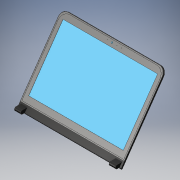
# Autodesk Inventor part: MONITOR
Saved by Autodesk Inventor 2025 (Build 290162000, 162)
## iProperties
Created: 2017-02-17
Part Number: MONITOR
Material: Generic
Document SubType Name: Modeling
Designer: Ali
Density: 1 g/cm^3
Appearance: Default
Author: Ali
Autodesk Inventor part; units mm, degrees
ref_plane "XZ Plane" through (0, 0, 0) normal (0, 1, 0) x (-1, 0, 0)
ref_plane "XY Plane" through (0, 0, 0) normal (0, 0, 1) x (1, 0, 0)
sketch "Sketch1" plane through (0, 0, 0) normal (0, 0, 1) x (1, 0, 0)
  line L0 (-145, 250) -> (145, 250)
  line L1 (165, 230) -> (165, 0)
  line L2 (165, 0) -> (-165, 0)
  line L3 (-165, 0) -> (-165, 230)
  arc A0 (-145, 250) -> (-165, 230) centre (-145, 230) ccw
  arc A1 (165, 230) -> (145, 250) centre (145, 230) ccw
  point P0 (0, 0)
  point P1 (165, 250)
  dimension "d2" = 330
  dimension "d3" = 250
  dimension "d4" = 20
  constraints: 8 end point, 4 point on circle, 4 tangent, 2 centre point, 2 parallel, 2 point on line, 1 equal radius, 1 horizontal, 1 perpendicular
  measures "d2" distance of L1.end L2.end
  measures "d3" distance of point (165, 250) L1.end
  measures "d4" radius of A0
extrude "MONITOR" add sketch "Sketch1" along normal blind 5
sketch "Sketch2" plane through (0, 0, 5) normal (0, 0, 1) x (1, 0, 0)
  line L0 (150, 40) -> (-150, 40)
  line L1 (-150, 40) -> (-150, 230)
  line L2 (-150, 230) -> (150, 230)
  line L3 (150, 230) -> (150, 40)
  dimension "d9" = 300
  dimension "d10" = 190
  constraints: 8 end point, 2 parallel, 1 horizontal, 1 perpendicular
  measures "d9" distance of L1.end L2.end
  measures "d10" distance of L0.end L1.end
extrude "SCREEN" cut sketch "Sketch2" against normal blind 0.5
sketch "Sketch3" plane through (0, 0, 5) normal (0, 0, 1) x (1, 0, 0)
  circle A0 centre (0, 240) radius 2.5
  point P0 (0, 0)
  constraints: 1 centre point
sketch "Sketch4" plane through (0, 240, 5.25) normal (0, 0, 1) x (1, 0, 0)
  point P0 (0, -240)
  point P1 (0, 0)
extrude "CAMERA" add sketch "Sketch3" along normal blind 0.25
extrude "CAMERA" add sketch "Sketch3" along normal blind 0.25
hole "CAMERA " at (0, 240, 5.25) direction (0, 0, -1) diameter 1 depth 0.1 tip angle 118
sketch "Sketch5" plane through (0, 0, 5) normal (0, 0, 1) x (1, 0, 0)
  point P0 (0, 0)
  point P1 (15, 240)
  point P2 (30, 240)
  point P3 (-15, 240)
hole "AESTHETICS" at (15, 240, 5) at (30, 240, 5) at (-15, 240, 5) direction (0, 0, -1) diameter 1 depth 0.1 tip angle 118
sketch "Sketch6" plane through (0, 0, 5) normal (0, 0, 1) x (1, 0, 0)
  line L0 (164.5, 20) -> (-164.5, 20)
  line L1 (-164.5, 20) -> (-164.5, 229)
  line L2 (-144, 249.5) -> (144, 249.5)
  line L3 (164.5, 229) -> (164.5, 20)
  arc A0 (-144, 249.5) -> (-164.5, 229) centre (-144, 229) ccw
  arc A1 (164.5, 229) -> (144, 249.5) centre (144, 229) ccw
  point P0 (-164.5, 249.5)
  point P1 (164.5, 249.5)
  dimension "d36" = 229.5
  dimension "d37" = 20.5
  dimension "d38" = 329
  constraints: 8 end point, 4 point on circle, 4 point on line, 4 tangent, 2 centre point, 2 parallel, 1 equal radius, 1 horizontal, 1 perpendicular
  measures "d36" distance of L0.end point (-164.5, 249.5)
  measures "d37" radius of A0
  measures "d38" distance of L0.start L0.end
extrude "SIDE BAND" add sketch "Sketch6" along normal blind 0.15
sketch "Sketch7" plane through (0, 0, 5) normal (0, 0, 1) x (1, 0, 0)
  line L0 (161.5, 23) -> (-161.5, 23)
  line L1 (-161.5, 23) -> (-161.5, 223)
  line L2 (-138, 246.5) -> (138, 246.5)
  line L3 (161.5, 223) -> (161.5, 23)
  arc A0 (-138, 246.5) -> (-161.5, 223) centre (-138, 223) ccw
  arc A1 (161.5, 223) -> (138, 246.5) centre (138, 223) ccw
  point P0 (-161.5, 246.5)
  point P1 (161.5, 246.5)
  dimension "d47" = 323
  dimension "d48" = 223.5
  dimension "d49" = 23.5
  constraints: 8 end point, 4 point on circle, 4 point on line, 4 tangent, 2 centre point, 2 parallel, 1 equal radius, 1 horizontal, 1 perpendicular
  measures "d47" distance of point (-161.5, 246.5) point (161.5, 246.5)
  measures "d48" distance of L0.end point (-161.5, 246.5)
  measures "d49" radius of A0
extrude "SIDE BAND 1" cut sketch "Sketch7" along normal blind 0.15
sketch "Sketch8" plane through (165, 0, 0) normal (1, 0, 0) x (0, 0, -1)
  line L0 (0, 0) -> (-5, 0)
  line L1 (-5, 0) -> (-5, 2.251)
  line L2 (-5, 2.251) -> (0, 2.251)
  line L3 (0, 2.251) -> (0, 0)
  constraints: 8 end point, 2 parallel, 1 horizontal, 1 perpendicular
extrude "CUT" cut sketch "Sketch8" against normal blind 330
sketch "Sketch9" plane through (165, 230, 5) normal (1, 0, 0) x (0, 0, -1)
  arc A0 (0, -227.749) -> (5, -227.749) centre (2.5, -227.749) ccw
  line L0 (0, -227.749) -> (5, -227.749)
  constraints: 2 end point, 2 point on circle, 1 centre point
extrude "ROUND BASE" add sketch "Sketch9" against normal blind 330
ref_plane "Work Plane1" through (150, 0, 0) normal (1, 0, 0) x (0, 1, 0)
sketch "Sketch10" plane through (150, 0, 0) normal (1, 0, 0) x (0, 1, 0)
  line L0 (2.2964, 5) -> (-2.2922, 11.5532)
  line L1 (2.2964, 5) -> (10.2964, 5) construction
  line L2 (2.2964, 5) -> (16.2964, 5)
  line L3 (16.2964, 5) -> (7.102, 18.1311)
  arc A0 (7.102, 18.1311) -> (-2.2922, 11.5532) centre (2.4049, 14.8421) ccw
  dimension "d58" = 8
  dimension "d60" = 14
  dimension "d62" = 16.0301
  dimension "d63" = 5.7341
  constraints: 8 end point, 2 point on circle, 1 centre point, 1 equal length, 1 horizontal
  measures "d58" distance of L0.end L0.start
  measures "d60" distance of L0.start L2.end
  measures "d62" distance of L2.end L3.end
  measures "d63" radius of A0
extrude "HINGE" add sketch "Sketch10" along normal mid plane 20
pattern_linear "HINGE 1" count 2 spacing 300 along (-1, 0, 0) of "HINGE"
move or copy body "Move Body1" bodies to move or copy 1 copy no rotation origin (0, 0, 0) rotation axis (1, 0, 0) rotation angle -35
move or copy body "Move Body2" bodies to move or copy 1 copy no translate (10, 0, 0)
body "Solid1"
